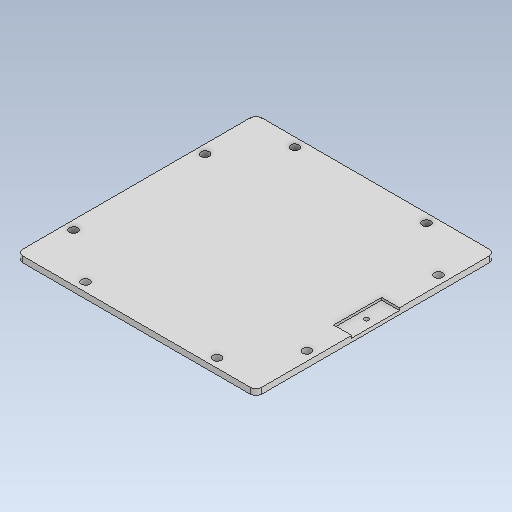
# Autodesk Inventor part: top_plate
Saved by Autodesk Inventor 2021 (Build 250183000, 183)
## iProperties
Created: 2020-07-18
Part Number: top_plate
Material: Generic
Document SubType Name: Modeling
Designer: Andrew
Density: 1 g/cm^3
Appearance: Default
Mass: 197.153 g
Surface Area: 842.381 cm^2
Volume: 197.153 cm^3
Author: Andrew
Autodesk Inventor part; units mm, degrees
ref_plane "YZ Plane" through (0, 0, 0) normal (1, 0, 0) x (0, 1, 0)
ref_plane "XZ Plane" through (0, 0, 0) normal (0, 1, 0) x (-1, 0, 0)
sketch "Sketch1" plane through (0, 0, 0) normal (0, 1, 0) x (-1, 0, 0)
  line L0 (0, 0) -> (200, 0)
  line L1 (200, 0) -> (200, -200)
  line L2 (200, -200) -> (0, -200)
  line L3 (0, -200) -> (0, 0)
  dimension "d0" = 200
  dimension "d1" = 200
  constraints: 8 end point, 2 parallel, 1 horizontal, 1 perpendicular
  measures "d0" distance of L1.end L2.end
  measures "d1" distance of L0.end L1.end
extrude "Extrusion1" add sketch "Sketch1" along normal blind 5
fillet "Fillet2" radius 5 4 edges at (0, 2.5, 0) (0, 2.5, -200) (-200, 2.5, 0) (-200, 2.5, -200)
sketch "Sketch4" plane through (0, 5, 0) normal (0, 1, 0) x (1, 0, 0)
  circle A0 centre (-7.5, 50) radius 3.5
  circle A1 centre (-40, 7.5) radius 3.5
  line L0 (-195, 0) -> (-5, 0) projected
  line L1 (0, 5) -> (0, 195) projected
  circle A2 centre (-150, 7.5) radius 3.5
  circle A3 centre (-192.5, 40) radius 3.5
  line L2 (-200, 195) -> (-200, 5) projected
  circle A4 centre (-192.5, 150) radius 3.5
  circle A5 centre (-160, 192.5) radius 3.5
  circle A6 centre (-50, 192.5) radius 3.5
  circle A7 centre (-7.5, 160) radius 3.5
  line L3 (-5, 200) -> (-195, 200) projected
  point P0 (0, 0)
  dimension "d42" = 7
  dimension "d43" = 7
  dimension "d44" = 50
  dimension "d45" = 40
  dimension "d46" = 7.5
  dimension "d47" = 7.5
  dimension "d48" = 7
  dimension "d49" = 7
  dimension "d50" = 40
  dimension "d51" = 50
  dimension "d52" = 7.5
  dimension "d53" = 7.5
  dimension "d73" = 7.5
  dimension "d74" = 7.5
  dimension "d75" = 7.5
  dimension "d76" = 7.5
  dimension "d77" = 7
  dimension "d78" = 7
  dimension "d79" = 7
  dimension "d80" = 7
  dimension "d81" = 50
  dimension "d82" = 40
  dimension "d83" = 50
  dimension "d84" = 40
  constraints: 8 centre point
  measures "d42" diameter of A0
  measures "d43" diameter of A1
  measures "d44" distance from line of L0 A0.centre
  measures "d45" distance from line of L1 A1.centre
  measures "d46" distance from line of L1 A0.centre
  measures "d47" distance from line of L0 A1.centre
  measures "d48" diameter of A2
  measures "d49" diameter of A3
  measures "d50" distance from line of L0 A3.centre
  measures "d51" distance from line of L2 A2.centre
  measures "d52" distance from line of L2 A3.centre
  measures "d53" distance from line of L0 A2.centre
  measures "d73" distance from line of L2 A4.centre
  measures "d74" distance from line of L3 A5.centre
  measures "d75" distance from line of L3 A6.centre
  measures "d76" distance from line of L1 A7.centre
  measures "d77" diameter of A4
  measures "d78" diameter of A5
  measures "d79" diameter of A6
  measures "d80" diameter of A7
  measures "d81" distance from line of L3 A4.centre
  measures "d82" distance from line of L2 A5.centre
  measures "d83" distance from line of L1 A6.centre
  measures "d84" distance from line of L3 A7.centre
extrude "Extrusion4" cut sketch "Sketch4" against normal through all
ref_plane "Work Plane2" through (-195, 0, -100) normal (0, 0, 1) x (1, 0, 0)
sketch "Sketch5" plane through (0, 5, 0) normal (0, 1, 0) x (1, 0, 0)
  line L0 (-195, 0) -> (-5, 0) projected
  line L1 (-5, 200) -> (-195, 200) projected
  line L2 (0, 120) -> (-15, 120)
  line L3 (-15, 120) -> (-15, 80)
  line L4 (-15, 80) -> (0, 80)
  line L5 (0, 80) -> (0, 120)
  line L6 (0, 5) -> (0, 195) projected
  point P0 (0, 0)
  dimension "d58" = 80
  dimension "d59" = 80
  dimension "d60" = 15
  dimension "d61" = 0
  constraints: 8 end point, 2 parallel, 1 horizontal, 1 perpendicular
  measures "d58" distance between parallel lines of L1 L2
  measures "d59" distance between parallel lines of L0 L4
  measures "d60" distance of L2.start L2.end
  measures "d61" distance between parallel lines of L6 L5
extrude "Extrusion5" cut sketch "Sketch5" against normal blind 2
sketch "Sketch6" plane through (0, 3, 0) normal (0, 1, 0) x (1, 0, 0)
  line L0 (0, 120) -> (0, 80) projected
  line L1 (0, 80) -> (-15, 80) projected
  point P0 (0, 0)
  point P1 (-7.5, 100)
  dimension "d64" = 7.5
  dimension "d65" = 20
  measures "d64" distance from line of point (-7.5, 100) L0
  measures "d65" distance from line of point (-7.5, 100) L1
hole "Hole1" at (-7.5, 3, -100) direction (0, -1, 0) diameter 4 end through all
body "Solid1"
